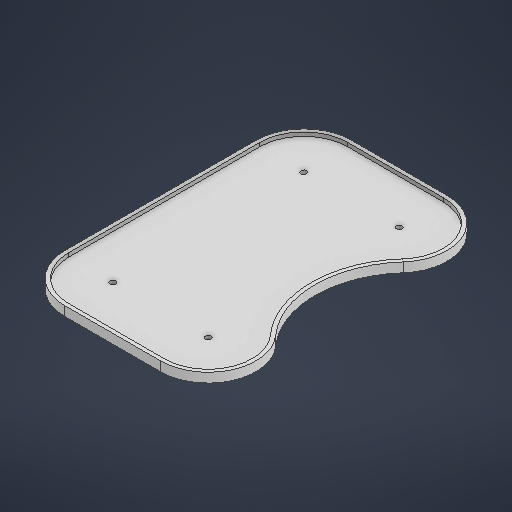
# Autodesk Inventor part: ControllerBottom
Saved by Autodesk Inventor 2026.1 (Build 301233000, 233)
## iProperties
Created: 2026-07-05
Part Number: ControllerBottom
Material: Generic
Document SubType Name: Modeling
Designer: Kasi Pusuluri
Density: 1 g/cm^3
Appearance: Default
Author: Kasi Pusuluri
Autodesk Inventor part; units mm, degrees
ref_plane "YZ Plane" through (0, 0, 0) normal (1, 0, 0) x (0, 1, 0)
ref_plane "XZ Plane" through (0, 0, 0) normal (0, 1, 0) x (-1, 0, 0)
ref_plane "XY Plane" through (0, 0, 0) normal (0, 0, 1) x (1, 0, 0)
sketch "Sketch1" plane through (0, 0, 0) normal (0, 1, 0) x (-1, 0, 0)
  line L0 (-25.4, 76.2) -> (25.4, 76.2)
  line L1 (-50.8, 50.8) -> (-50.8, -50.8)
  line L2 (50.8, 76.2) -> (-50.8, 76.2)
  line L3 (-25.4, -76.2) -> (25.4, -76.2)
  line L4 (50.8, -50.8) -> (50.8, 50.8)
  arc A0 (50.8, 50.8) -> (25.4, 76.2) centre (25.4, 50.8) ccw
  arc A1 (25.4, -76.2) -> (50.8, -50.8) centre (25.4, -50.8) ccw
  arc A2 (-50.8, -50.8) -> (-25.4, -76.2) centre (-25.4, -50.8) ccw
  arc A3 (-25.4, 76.2) -> (-50.8, 50.8) centre (-25.4, 50.8) ccw
  circle A4 centre (-25.4, 50.8) radius 25.4
  circle A5 centre (-25.4, -50.8) radius 25.4
  circle A6 centre (-50.8, 0) radius 31.3961
  circle A7 centre (-82.1961, 0) radius 50.8
  point P0 (-36.7592, 28.0815)
  point P1 (-36.7592, -28.0815)
  point P2 (-50.8, 31.3961)
  point P3 (-50.8, -31.3961)
  point P4 (-44.332, 33.8667)
  point P5 (-44.332, -33.8667)
  dimension "d6" = 101.6
  dimension "d21" = 25.4
  constraints: 10 end point, 9 tangent, 8 point on circle, 7 centre point, 6 coincident, 4 equal radius, 3 point on line, 2 horizontal, 1 parallel, 4 other
  measures "d6" distance of point (-50.8, 76.2) L2.start
  measures "d21" radius of A0
extrude "Extrusion5" add sketch "Sketch1" along normal blind 3 contours A4 A3 | L0 A0 L4 A1 L3 A5 A6 A4 | A4 A6 A7 | A6 A7 | A5 A2 | A7 A6 A5
sketch "Sketch3" plane through (0, 3, 0) normal (0, 1, 0) x (1, 0, 0)
  arc A0 (-50.8, -50.8) -> (-25.4, -76.2) centre (-25.4, -50.8) ccw projected
  arc A1 (-50.8, -50.8) -> (-25.4, -76.2) centre (-25.4, -50.8) ccw
  arc A2 (-25.4, 76.2) -> (-50.8, 50.8) centre (-25.4, 50.8) ccw projected
  line L0 (-50.8, 50.8) -> (-50.8, -50.8) projected
  arc A3 (-25.4, 76.2) -> (-50.8, 50.8) centre (-25.4, 50.8) ccw
  arc A4 (25.4, -76.2) -> (44.332, -33.8667) centre (25.4, -50.8) ccw projected
  arc A5 (25.4, -76.2) -> (44.332, -33.8667) centre (25.4, -50.8) ccw
  arc A6 (44.332, 33.8667) -> (44.332, -33.8667) centre (82.1961, 0) ccw projected
  arc A7 (44.332, 33.8667) -> (44.332, -33.8667) centre (82.1961, 0) ccw
  arc A8 (44.332, 33.8667) -> (25.4, 76.2) centre (25.4, 50.8) ccw projected
  arc A9 (44.332, 33.8667) -> (25.4, 76.2) centre (25.4, 50.8) ccw
  line L1 (-50.8, -50.8) -> (-50.8, 50.8)
  line L2 (-25.4, -76.2) -> (25.4, -76.2) projected
  line L3 (-25.4, -76.2) -> (25.4, -76.2)
  line L4 (-25.4, 76.2) -> (25.4, 76.2)
  line L5 (-25.4, 76.2) -> (25.4, 76.2)
  line L6 (25.4, 76.2) -> (-25.4, 76.2)
  line L7 (25.4, 76.2) -> (-25.4, 76.2) projected
  line L8 (25.4, 76.2) -> (-25.4, 76.2)
  arc A10 (-48.8, -50.8) -> (-25.4, -74.2) centre (-25.4, -50.8) ccw
  line L9 (-25.4, -74.2) -> (25.4, -74.2)
  arc A11 (25.4, -74.2) -> (42.8413, -35.2) centre (25.4, -50.8) ccw
  arc A12 (42.8413, 35.2) -> (42.8413, -35.2) centre (82.1961, 0) ccw
  arc A13 (42.8413, 35.2) -> (25.4, 74.2) centre (25.4, 50.8) ccw
  line L10 (25.4, 74.2) -> (-25.4, 74.2)
  arc A14 (-25.4, 74.2) -> (-48.8, 50.8) centre (-25.4, 50.8) ccw
  line L11 (-48.8, 50.8) -> (-48.8, -50.8)
  point P0 (0, 0)
  dimension "d28" = 2
  constraints: 23 point on circle, 18 end point, 10 centre point, 3 horizontal, 2 collinear, 2 concentric, 1 tangent, 7 other
  measures "d28" distance between parallel lines of L11 L0
extrude "Extrusion6" add sketch "Sketch3" along normal blind 2
hole "Hole2" at (-25.4, 0, 50.8) at (25.4, 0, 50.8) at (25.4, 0, -50.8) at (-25.4, 0, -50.8) direction (0, 1, 0) diameter 3 depth 25.4 tip angle 118
body "Solid5"
